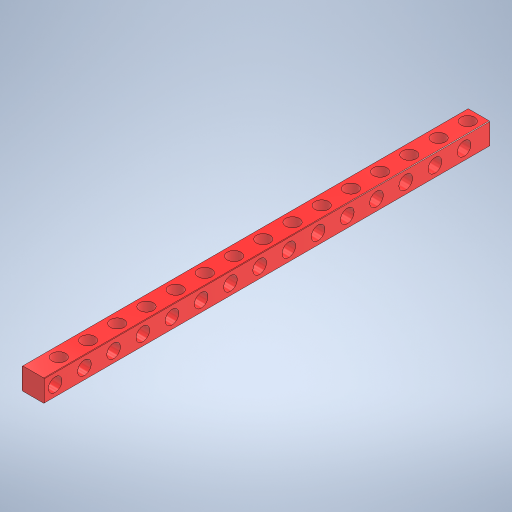
# Autodesk Inventor part: Nut Strip
Saved by Autodesk Inventor 2023.2 (Build 272271000, 271)
## iProperties
Created: 2024-01-21
Part Number: Nut Strip
Material: Aluminum 6061
Document SubType Name: Modeling
Designer: Nathan Cai
Density: 2.7 g/cm^3
Appearance: Light Red
Author: Nathan Cai
Autodesk Inventor part; units mm, degrees
ref_plane "YZ Plane" through (0, 0, 0) normal (1, 0, 0) x (0, 1, 0)
ref_plane "XZ Plane" through (0, 0, 0) normal (0, 1, 0) x (-1, 0, 0)
ref_plane "XY Plane" through (0, 0, 0) normal (0, 0, 1) x (1, 0, 0)
sketch "Sketch1" plane through (0, 0, 0) normal (0, 0, 1) x (1, 0, 0)
  line L0 (-2.3812, -2.3813) -> (2.3813, -2.3813)
  line L1 (2.3813, -2.3813) -> (2.3812, 2.3812)
  line L2 (2.3812, 2.3812) -> (-2.3813, 2.3812)
  line L3 (-2.3813, 2.3812) -> (-2.3812, -2.3813)
  line L4 (-2.3812, -2.3813) -> (2.3812, 2.3812) construction
  line L5 (2.3813, -2.3813) -> (-2.3813, 2.3812) construction
  point P0 (0, 0)
  dimension "d0" = 4.7625
  dimension "d1" = 4.7625
  constraints: 12 end point, 2 midpoint, 2 parallel, 1 horizontal, 1 perpendicular
  measures "d0" distance of L2.end L1.end
  measures "d1" distance of L1.end L0.end
extrude "Extrusion1" add sketch "Sketch1" along normal blind 96.8375
sketch "Sketch2" plane through (-2.3813, 2.3812, 0) normal (0, 1, 0) x (1, 0, 0)
  line L0 (2.3813, 0) -> (2.3813, -96.8375) construction
  line L1 (4.7625, -96.8375) -> (0, -96.8375) projected
  circle A0 centre (2.3813, -2.3813) radius 1.4732
  circle A1 centre (2.3813, -8.7313) radius 1.4732
  circle A2 centre (2.3813, -15.0813) radius 1.4732
  circle A3 centre (2.3813, -21.4313) radius 1.4732
  circle A4 centre (2.3813, -26.1938) radius 1.4493 construction
  line L2 (4.7625, 0) -> (0, 0) projected
  circle A5 centre (2.3813, -27.7812) radius 1.4732
  circle A6 centre (2.3813, -34.1313) radius 1.4732
  circle A7 centre (2.3813, -40.4812) radius 1.4732
  circle A8 centre (2.3813, -46.8313) radius 1.4732
  circle A9 centre (2.3813, -53.1813) radius 1.4732
  circle A10 centre (2.3813, -59.5312) radius 1.4732
  circle A11 centre (2.3813, -65.8812) radius 1.4732
  circle A12 centre (2.3813, -72.2313) radius 1.4732
  circle A13 centre (2.3813, -78.5812) radius 1.4732
  circle A14 centre (2.3813, -84.9313) radius 1.4732
  circle A15 centre (2.3813, -91.2812) radius 1.4732
  dimension "d4" = 2.9464
  dimension "d7" = 6.35
  dimension "d12" = 4.7625
  dimension "d13" = 2.3813
  constraints: 16 centre point, 2 end point, 2 point on line, 1 midpoint, 1 vertical, 28 other
  measures "d4" diameter of A0
  measures "d7" distance of A0.centre A1.centre
  measures "d12" distance of A3.centre A4.centre
  measures "d13" distance from line of L2 A0.centre
extrude "Extrusion2" cut sketch "Sketch2" against normal through all
sketch "Sketch3" plane through (2.3813, -2.3813, 0) normal (1, 0, 0) x (0, 0, -1)
  line L0 (0, 2.3813) -> (-96.8375, 2.3813) construction
  line L1 (-96.8375, 0) -> (-96.8375, 4.7625) projected
  circle A0 centre (-94.4562, 2.3813) radius 1.4732
  circle A1 centre (-88.1063, 2.3813) radius 1.4732
  circle A2 centre (-81.7562, 2.3813) radius 1.4732
  circle A3 centre (-75.4062, 2.3813) radius 1.4732
  circle A4 centre (-69.0562, 2.3813) radius 1.4732
  circle A5 centre (-62.7062, 2.3813) radius 1.4732
  circle A6 centre (-56.3562, 2.3813) radius 1.4732
  circle A7 centre (-50.0062, 2.3813) radius 1.4732
  circle A8 centre (-43.6562, 2.3813) radius 1.4732
  circle A9 centre (-37.3062, 2.3813) radius 1.4732
  circle A10 centre (-30.9563, 2.3813) radius 1.4732
  circle A11 centre (-24.6062, 2.3813) radius 1.4732
  circle A12 centre (-18.2562, 2.3813) radius 1.4732
  circle A13 centre (-11.9062, 2.3813) radius 1.4732
  circle A14 centre (-5.5562, 2.3813) radius 1.4732
  dimension "d16" = 2.9464
  dimension "d17" = 2.3813
  dimension "d20" = 6.35
  constraints: 15 centre point, 2 end point, 1 horizontal, 1 midpoint, 1 point on line, 28 other
  measures "d16" diameter of A0
  measures "d17" distance from line of L1 A0.centre
  measures "d20" distance of A0.centre A1.centre
extrude "Extrusion3" cut sketch "Sketch3" against normal through all
chamfer "Chamfer1" distance 0.1 angle 45 4 edges at (-2.3813, 2.3812, 48.4188) (2.3812, 2.3812, 48.4188) (2.3813, -2.3813, 48.4188) (-2.3812, -2.3813, 48.4188)
equation "\"d1\" = d0"
body "Solid1"
